Autodesk Inventor part; units mm, degrees
(part 3 of 6)
sketch "Sketch39" plane through (0, 0, 35) normal (0, 0, 1) x (1, 0, 0)
  line L0 (24.1, -52.4001) -> (24.1, -46.4001) projected
  line L1 (24.1, -90.2001) -> (30.1, -90.2001) projected
  line L2 (30.1, -46.4001) -> (30.1, -52.4001) projected
  line L3 (30.1, -96.2001) -> (24.1, -96.2001) projected
  line L4 (-30.1, -46.4001) -> (-24.1, -46.4001) projected
  line L5 (-24.1, -46.4001) -> (-24.1, -52.4001) projected
  line L6 (-24.1, -52.4001) -> (-30.1, -52.4001) projected
  line L7 (-30.1, -52.4001) -> (-30.1, -46.4001) projected
  line L8 (-30.1, -90.2001) -> (-24.1, -90.2001) projected
  line L9 (-24.1, -96.2001) -> (-30.1, -96.2001) projected
  line L10 (24.1, -46.4001) -> (30.1, -46.4001) projected
  line L11 (30.1, -52.4001) -> (24.1, -52.4001) projected
  line L12 (-44.1, -54.2001) -> (44.1, -54.2001) projected
  arc A0 (44.1, -64.2001) -> (44.1, -54.2001) centre (44.1, -59.2001) ccw projected
  line L13 (44.1, -64.2001) -> (44.1, -78.4001) projected
  arc A1 (44.1, -88.4001) -> (44.1, -78.4001) centre (44.1, -83.4001) ccw projected
  line L14 (44.1, -88.4001) -> (-44.1, -88.4001) projected
  line L15 (-44.1, -88.4001) -> (-44.1, -54.2001) projected
  line L16 (-103.1549, -6.3815) -> (-96.791, -0.0176) projected
  line L17 (-96.791, -0.0176) -> (-95.5889, 1.1845) projected
  line L18 (-95.5889, 1.1845) -> (-91.3463, -3.0581) projected
  line L19 (-91.3463, -3.0581) -> (-75.0828, -19.3216) projected
  line L20 (-75.0828, -19.3216) -> (-71.5473, -22.8571) projected
  line L21 (-71.5473, -22.8571) -> (-80.3154, -31.6252) projected
  line L22 (-80.3154, -31.6252) -> (-83.8509, -28.0897) projected
  line L23 (-83.8509, -28.0897) -> (-100.1144, -11.8263) projected
  line L24 (-100.1144, -11.8263) -> (-104.357, -7.5836) projected
  line L25 (-104.357, -7.5836) -> (-103.1549, -6.3815) projected
  line L26 (4.5, -160.1002) -> (-4.5, -160.1002) projected
  line L27 (-4.5, -160.1002) -> (-6.2, -160.1002) projected
  line L28 (-6.2, -160.1002) -> (-6.2, -154.1002) projected
  line L29 (-6.2, -154.1002) -> (-6.2, -131.1002) projected
  line L30 (-6.2, -131.1002) -> (-6.2, -126.1002) projected
  line L31 (-6.2, -126.1002) -> (6.2, -126.1002) projected
  line L32 (6.2, -126.1002) -> (6.2, -131.1002) projected
  line L33 (6.2, -131.1002) -> (6.2, -154.1002) projected
  line L34 (6.2, -154.1002) -> (6.2, -160.1002) projected
  line L35 (6.2, -160.1002) -> (4.5, -160.1002) projected
  line L36 (96.791, -0.0176) -> (103.1549, -6.3815) projected
  line L37 (103.1549, -6.3815) -> (104.357, -7.5836) projected
  line L38 (104.357, -7.5836) -> (100.1144, -11.8263) projected
  line L39 (100.1144, -11.8263) -> (83.8509, -28.0897) projected
  line L40 (83.8509, -28.0897) -> (80.3154, -31.6252) projected
  line L41 (80.3154, -31.6252) -> (71.5473, -22.8571) projected
  line L42 (71.5473, -22.8571) -> (75.0828, -19.3216) projected
  line L43 (75.0828, -19.3216) -> (91.3463, -3.0581) projected
  line L44 (91.3463, -3.0581) -> (95.5889, 1.1845) projected
  line L45 (95.5889, 1.1845) -> (96.791, -0.0176) projected
  line L46 (76.8724, -48.8001) -> (88.2822, -48.8001) projected
  line L47 (88.2822, -48.8001) -> (94.3529, -27.4901) projected
  line L48 (94.3529, -27.4901) -> (106.8333, -15.0097) projected
  arc A2 (106.8333, -15.0097) -> (88.1629, 3.6608) centre (97.4981, -5.6744) ccw projected
  line L49 (88.1629, 3.6608) -> (75.6824, -8.8196) projected
  line L50 (75.6824, -8.8196) -> (57.202, -21.3001) projected
  line L51 (57.202, -21.3001) -> (38.202, -31.3001) projected
  line L52 (38.202, -31.3001) -> (19.202, -21.3001) projected
  line L53 (19.202, -21.3001) -> (13.202, -3.65) projected
  line L54 (13.202, -3.65) -> (13.202, 14) projected
  arc A3 (13.202, 14) -> (-13.202, 14) centre (0, 14) ccw projected
  line L55 (-13.202, 14) -> (-13.202, -3.65) projected
  line L56 (-13.202, -3.65) -> (-19.202, -21.3001) projected
  line L57 (-19.202, -21.3001) -> (-38.202, -31.3001) projected
  line L58 (-38.202, -31.3001) -> (-57.202, -21.3001) projected
  line L59 (-57.202, -21.3001) -> (-75.6824, -8.8196) projected
  line L60 (-75.6824, -8.8196) -> (-88.1629, 3.6608) projected
  arc A4 (-88.1629, 3.6608) -> (-106.8333, -15.0097) centre (-97.4981, -5.6744) ccw projected
  line L61 (-106.8333, -15.0097) -> (-94.3529, -27.4901) projected
  line L62 (-94.3529, -27.4901) -> (-76.3482, -71.3001) projected
  line L63 (-76.3482, -71.3001) -> (-94.3529, -115.1101) projected
  line L64 (-94.3529, -115.1101) -> (-106.8333, -127.5905) projected
  arc A5 (-106.8333, -127.5905) -> (-88.1629, -146.2609) centre (-97.4981, -136.9257) ccw projected
  line L65 (-88.1629, -146.2609) -> (-75.6824, -133.7805) projected
  line L66 (-75.6824, -133.7805) -> (-57.202, -121.3001) projected
  line L67 (-57.202, -121.3001) -> (-38.202, -111.3001) projected
  line L68 (-38.202, -111.3001) -> (-19.202, -121.3001) projected
  line L69 (-19.202, -121.3001) -> (-13.202, -138.9501) projected
  line L70 (-13.202, -138.9501) -> (-13.202, -156.6002) projected
  arc A6 (-13.202, -156.6002) -> (13.202, -156.6002) centre (0, -156.6002) ccw projected
  line L71 (13.202, -156.6002) -> (13.202, -138.9501) projected
  line L72 (13.202, -138.9501) -> (19.202, -121.3001) projected
  line L73 (19.202, -121.3001) -> (38.202, -111.3001) projected
  line L74 (38.202, -111.3001) -> (57.202, -121.3001) projected
  line L75 (57.202, -121.3001) -> (75.6824, -133.7805) projected
  line L76 (75.6824, -133.7805) -> (88.1629, -146.2609) projected
  arc A7 (88.1629, -146.2609) -> (106.8333, -127.5905) centre (97.4981, -136.9257) ccw projected
  line L77 (106.8333, -127.5905) -> (94.3529, -115.1101) projected
  line L78 (94.3529, -115.1101) -> (88.2822, -93.8001) projected
  line L79 (88.2822, -93.8001) -> (76.8724, -93.8001) projected
  line L80 (76.8724, -93.8001) -> (76.8724, -48.8001) projected
  line L81 (-96.791, -142.5826) -> (-103.1549, -136.2186) projected
  line L82 (-103.1549, -136.2186) -> (-104.357, -135.0165) projected
  line L83 (-104.357, -135.0165) -> (-100.1144, -130.7739) projected
  line L84 (-100.1144, -130.7739) -> (-83.8509, -114.5104) projected
  line L85 (-83.8509, -114.5104) -> (-80.3154, -110.9749) projected
  line L86 (-80.3154, -110.9749) -> (-71.5473, -119.743) projected
  line L87 (-71.5473, -119.743) -> (-75.0828, -123.2786) projected
  line L88 (-75.0828, -123.2786) -> (-91.3463, -139.542) projected
  line L89 (-91.3463, -139.542) -> (-95.5889, -143.7847) projected
  line L90 (-95.5889, -143.7847) -> (-96.791, -142.5826) projected
  line L91 (103.1549, -136.2186) -> (96.791, -142.5826) projected
  line L92 (96.791, -142.5826) -> (95.5889, -143.7847) projected
  line L93 (95.5889, -143.7847) -> (91.3463, -139.542) projected
  line L94 (91.3463, -139.542) -> (75.0828, -123.2786) projected
  line L95 (75.0828, -123.2786) -> (71.5473, -119.743) projected
  line L96 (71.5473, -119.743) -> (80.3154, -110.9749) projected
  line L97 (80.3154, -110.9749) -> (83.8509, -114.5104) projected
  line L98 (83.8509, -114.5104) -> (100.1144, -130.7739) projected
  line L99 (100.1144, -130.7739) -> (104.357, -135.0165) projected
  line L100 (104.357, -135.0165) -> (103.1549, -136.2186) projected
  line L101 (-4.5, 17.5) -> (4.5, 17.5) projected
  line L102 (4.5, 17.5) -> (6.2, 17.5) projected
  line L103 (6.2, 17.5) -> (6.2, 11.5) projected
  line L104 (6.2, 11.5) -> (6.2, -11.5) projected
  line L105 (6.2, -11.5) -> (6.2, -16.5) projected
  line L106 (6.2, -16.5) -> (-6.2, -16.5) projected
  line L107 (-6.2, -16.5) -> (-6.2, -11.5) projected
  line L108 (-6.2, -11.5) -> (-6.2, 11.5) projected
  line L109 (-6.2, 11.5) -> (-6.2, 17.5) projected
  line L110 (-6.2, 17.5) -> (-4.5, 17.5) projected
  circle A8 centre (-27.1, -93.2001) radius 1.5
  circle A9 centre (-27.1, -49.4001) radius 1.5
  circle A10 centre (27.1, -93.2001) radius 1.5
  circle A11 centre (27.1, -49.4001) radius 1.5
  line L111 (30.1, -90.2001) -> (30.1, -96.2001) projected
  line L112 (24.1, -96.2001) -> (24.1, -90.2001) projected
  line L113 (-30.1, -96.2001) -> (-30.1, -90.2001) projected
  line L114 (-24.1, -90.2001) -> (-24.1, -96.2001) projected
  point P0 (0, 0)
  dimension "d566" = 3
  dimension "d567" = 3
  dimension "d568" = 3
  dimension "d569" = 3
  dimension "d570" = 3
  dimension "d571" = 3
  dimension "d572" = 3
  dimension "d575" = 3
  dimension "d576" = 3
  dimension "d577" = 3
  constraints: 4 centre point
  measures "d566" diameter of A8
  measures "d567" diameter of A9
  measures "d568" diameter of A10
  measures "d569" diameter of A11
  measures "d570" distance from line of L1 A10.centre
  measures "d571" distance from line of L10 A11.centre
  measures "d572" distance from line of L2 A10.centre
  measures "d575" distance from line of L8 A8.centre
  measures "d576" distance from line of L5 A9.centre
  measures "d577" distance from line of L4 A9.centre
extrude "Extrusion39" cut sketch "Sketch39" against normal blind 100 contours A8 | A9 | A10 | A11
sketch "Sketch40" plane through (0, 0, -5) normal (0, 0, -1) x (-1, 0, 0)
  circle A0 centre (-27.1, -49.4001) radius 1.5 projected
  circle A1 centre (-27.1, -93.2001) radius 1.5 projected
  circle A2 centre (27.1, -49.4001) radius 1.5 projected
  circle A3 centre (27.1, -93.2001) radius 1.5 projected
  line L0 (-3.1216, -126.8818) -> (-0.0216, -125.092) projected
  line L1 (-0.0216, -125.092) -> (3.0784, -126.8818) projected
  line L2 (3.0784, -126.8818) -> (3.0784, -130.4614) projected
  line L3 (3.0784, -130.4614) -> (-0.0216, -132.2511) projected
  line L4 (-0.0216, -132.2511) -> (-3.1216, -130.4614) projected
  line L5 (-3.1216, -130.4614) -> (-3.1216, -126.8818) projected
  line L6 (-3.2524, -13.9963) -> (-1.6252, -11.1823) projected
  line L7 (-1.6252, -11.1823) -> (1.6252, -11.1846) projected
  line L8 (1.6252, -11.1846) -> (3.2486, -14.0007) projected
  line L9 (3.2486, -14.0007) -> (1.6214, -16.8146) projected
  line L10 (1.6214, -16.8146) -> (-1.6291, -16.8124) projected
  line L11 (-1.6291, -16.8124) -> (-3.2524, -13.9963) projected
  line L12 (-76.9445, -120.8328) -> (-80.5331, -119.7332) projected
  line L13 (-80.5331, -119.7332) -> (-81.3752, -116.0755) projected
  line L14 (-81.3752, -116.0755) -> (-78.6286, -113.5175) projected
  line L15 (-78.6286, -113.5175) -> (-75.0399, -114.6171) projected
  line L16 (-75.0399, -114.6171) -> (-74.1979, -118.2748) projected
  line L17 (-74.1979, -118.2748) -> (-76.9445, -120.8328) projected
  line L18 (74.0578, -118.2007) -> (74.9468, -114.5542) projected
  line L19 (74.9468, -114.5542) -> (78.5493, -113.5008) projected
  line L20 (78.5493, -113.5008) -> (81.2629, -116.094) projected
  line L21 (81.2629, -116.094) -> (80.3739, -119.7405) projected
  line L22 (80.3739, -119.7405) -> (76.7714, -120.7939) projected
  line L23 (76.7714, -120.7939) -> (74.0578, -118.2007) projected
  line L24 (81.3332, -26.5207) -> (78.6197, -29.1139) projected
  line L25 (78.6197, -29.1139) -> (75.0172, -28.0605) projected
  line L26 (75.0172, -28.0605) -> (74.1282, -24.4139) projected
  line L27 (74.1282, -24.4139) -> (76.8417, -21.8207) projected
  line L28 (76.8417, -21.8207) -> (80.4442, -22.8741) projected
  line L29 (80.4442, -22.8741) -> (81.3332, -26.5207) projected
  line L30 (-76.9117, -21.8446) -> (-74.165, -24.4027) projected
  line L31 (-74.165, -24.4027) -> (-75.0071, -28.0604) projected
  line L32 (-75.0071, -28.0604) -> (-78.5957, -29.16) projected
  line L33 (-78.5957, -29.16) -> (-81.3424, -26.6019) projected
  line L34 (-81.3424, -26.6019) -> (-80.5003, -22.9442) projected
  line L35 (-80.5003, -22.9442) -> (-76.9117, -21.8446) projected
  circle A4 centre (-91.4877, -11.6848) radius 5 projected
  circle A5 centre (0, -148.1002) radius 5 projected
  circle A6 centre (91.4877, -11.6848) radius 5 projected
  circle A7 centre (91.4877, -130.9153) radius 5 projected
  circle A8 centre (-91.4877, -130.9153) radius 5 projected
  circle A9 centre (0, 5.5) radius 5 projected
  line L36 (-13.202, -3.65) -> (-19.202, -21.3001) projected
  line L37 (-19.202, -21.3001) -> (-38.202, -31.3001) projected
  line L38 (-38.202, -31.3001) -> (-57.202, -21.3001) projected
  line L39 (-57.202, -21.3001) -> (-75.6824, -8.8196) projected
  line L40 (-75.6824, -8.8196) -> (-88.1629, 3.6608) projected
  arc A10 (-88.1629, 3.6608) -> (-106.8333, -15.0097) centre (-97.4981, -5.6744) ccw projected
  line L41 (-106.8333, -15.0097) -> (-94.3529, -27.4901) projected
  line L42 (-94.3529, -27.4901) -> (-81.8724, -71.3001) projected
  line L43 (-81.8724, -71.3001) -> (-94.3529, -115.1101) projected
  line L44 (-94.3529, -115.1101) -> (-106.8333, -127.5905) projected
  arc A11 (-106.8333, -127.5905) -> (-88.1629, -146.2609) centre (-97.4981, -136.9257) ccw projected
  line L45 (-88.1629, -146.2609) -> (-75.6824, -133.7805) projected
  line L46 (-75.6824, -133.7805) -> (-57.202, -121.3001) projected
  line L47 (-57.202, -121.3001) -> (-38.202, -111.3001) projected
  line L48 (-38.202, -111.3001) -> (-19.202, -121.3001) projected
  line L49 (-19.202, -121.3001) -> (-13.202, -138.9501) projected
  line L50 (-13.202, -138.9501) -> (-13.202, -156.6002) projected
  arc A12 (-13.202, -156.6002) -> (13.202, -156.6002) centre (0, -156.6002) ccw projected
  line L51 (13.202, -156.6002) -> (13.202, -138.9501) projected
  line L52 (13.202, -138.9501) -> (19.202, -121.3001) projected
  line L53 (19.202, -121.3001) -> (38.202, -111.3001) projected
  line L54 (38.202, -111.3001) -> (57.202, -121.3001) projected
  line L55 (57.202, -121.3001) -> (75.6824, -133.7805) projected
  line L56 (75.6824, -133.7805) -> (88.1629, -146.2609) projected
  arc A13 (88.1629, -146.2609) -> (106.8333, -127.5905) centre (97.4981, -136.9257) ccw projected
  line L57 (106.8333, -127.5905) -> (94.3529, -115.1101) projected
  line L58 (94.3529, -115.1101) -> (76.3482, -71.3001) projected
  line L59 (76.3482, -71.3001) -> (94.3529, -27.4901) projected
  line L60 (94.3529, -27.4901) -> (106.8333, -15.0097) projected
  arc A14 (106.8333, -15.0097) -> (88.1629, 3.6608) centre (97.4981, -5.6744) ccw projected
  line L61 (88.1629, 3.6608) -> (75.6824, -8.8196) projected
  line L62 (75.6824, -8.8196) -> (57.202, -21.3001) projected
  line L63 (57.202, -21.3001) -> (38.202, -31.3001) projected
  line L64 (38.202, -31.3001) -> (19.202, -21.3001) projected
  line L65 (19.202, -21.3001) -> (13.202, -3.65) projected
  line L66 (13.202, -3.65) -> (13.202, 14) projected
  arc A15 (13.202, 14) -> (-13.202, 14) centre (0, 14) ccw projected
  line L67 (-13.202, 14) -> (-13.202, -3.65) projected
  line L68 (25.3102, -96.3001) -> (23.5204, -93.2001)
  line L69 (23.5204, -93.2001) -> (25.3102, -90.1001)
  line L70 (25.3102, -90.1001) -> (28.8898, -90.1001)
  line L71 (28.8898, -90.1001) -> (30.6796, -93.2001)
  line L72 (30.6796, -93.2001) -> (28.8898, -96.3001)
  line L73 (28.8898, -96.3001) -> (25.3102, -96.3001)
  line L74 (-28.8898, -90.1001) -> (-25.3102, -90.1001)
  line L75 (-25.3102, -90.1001) -> (-23.5204, -93.2001)
  line L76 (-23.5204, -93.2001) -> (-25.3102, -96.3001)
  line L77 (-25.3102, -96.3001) -> (-28.8898, -96.3001)
  line L78 (-28.8898, -96.3001) -> (-30.6796, -93.2001)
  line L79 (-30.6796, -93.2001) -> (-28.8898, -90.1001)
  line L80 (-28.8898, -52.5001) -> (-30.6796, -49.4001)
  line L81 (-30.6796, -49.4001) -> (-28.8898, -46.3001)
  line L82 (-28.8898, -46.3001) -> (-25.3102, -46.3001)
  line L83 (-25.3102, -46.3001) -> (-23.5204, -49.4001)
  line L84 (-23.5204, -49.4001) -> (-25.3102, -52.5001)
  line L85 (-25.3102, -52.5001) -> (-28.8898, -52.5001)
  line L86 (25.3102, -52.5001) -> (23.5204, -49.4001)
  line L87 (23.5204, -49.4001) -> (25.3102, -46.3001)
  line L88 (25.3102, -46.3001) -> (28.8898, -46.3001)
  line L89 (28.8898, -46.3001) -> (30.6796, -49.4001)
  line L90 (30.6796, -49.4001) -> (28.8898, -52.5001)
  line L91 (28.8898, -52.5001) -> (25.3102, -52.5001)
  line L92 (-3.1216, -126.8818) -> (-0.0216, -125.092) projected
  line L93 (-0.0216, -125.092) -> (3.0784, -126.8818) projected
  point P0 (0, 0)
  dimension "d580" = 3.1
  dimension "d581" = 3.1
  dimension "d582" = 3.1
  dimension "d583" = 3.1
  constraints: 48 end point, 4 coincident, 4 perpendicular, 52 other
  measures "d580" distance from line of L76 A1.centre
  measures "d581" distance from line of L69 A3.centre
  measures "d582" distance from line of L91 A2.centre
  measures "d583" distance from line of L82 A0.centre
extrude "Extrusion40" cut sketch "Sketch40" against normal blind 2.4 contours A0 | A1 | A2 | A3 | L68 L69 L70 L71 L72 L73 | L74 L75 L76 L77 L78 L79 | L80 L81 L82 L83 L84 L85 | L86 L87 L88 L89 L90 L91
sketch "Sketch41" plane through (76.8724, -93.8001, 10) normal (-1, 0, 0) x (0, 0, 1)
  arc A0 (2.2, 18.95) -> (6.3, 18.95) centre (4.25, 18.95) ccw projected
  line L0 (2.2, 18.95) -> (2.2, 25.95) projected
  arc A1 (6.3, 25.95) -> (2.2, 25.95) centre (4.25, 25.95) ccw projected
  line L1 (6.3, 25.95) -> (6.3, 18.95) projected
  line L2 (0, 0) -> (0, 45) projected
  line L3 (0, 0) -> (25, 0) projected
  line L4 (25, 45) -> (25, 0) projected
  line L5 (0, 45) -> (25, 45) projected
  circle A2 centre (20.5, 43.45) radius 1
  circle A3 centre (20.5, 1.45) radius 1
  circle A4 centre (3.5, 1.45) radius 1
  circle A5 centre (3.5, 43.45) radius 1
  circle A6 centre (12, 35.95) radius 8
  circle A7 centre (12, 8.95) radius 8
  circle A8 centre (12, 35.95) radius 8.15
  circle A9 centre (12, 8.95) radius 8.15
  point P0 (-10, 93.8001)
  dimension "d586" = 0.15
  dimension "d587" = 0.15
  constraints: 8 centre point, 12 other
  measures "d586" radial gap between concentric circles of A8 A6
  measures "d587" radial gap between concentric circles of A9 A7
extrude "Extrusion41" cut sketch "Sketch41" against normal blind 20 contours A2 | A3 | A4 | A5 | A6 | A7 | A8 | A9
ref_plane "Work Plane1" through (88.2822, -48.8001, 10) normal (1, 0, 0) x (0, 0, 1)
sketch "Sketch42" plane through (88.2822, -48.8001, 10) normal (1, 0, 0) x (0, 0, 1)
  circle A0 centre (20.5, 43.55) radius 1 projected
  circle A1 centre (12, 36.05) radius 8.15 projected
  circle A2 centre (3.5, 43.55) radius 1 projected
  line L0 (25, 22.5) -> (-15, 22.5) projected
  line L1 (25, 45) -> (25, 22.5) projected
  line L2 (0, 45) -> (25, 45) projected
  line L3 (0, 66.31) -> (0, 45) projected
  line L4 (-15, 66.31) -> (0, 66.31) projected
  line L5 (-15, 22.5) -> (-15, 66.31) projected
  circle A3 centre (12, 9.05) radius 8.15 projected
  circle A4 centre (3.5, 1.55) radius 1 projected
  circle A5 centre (20.5, 1.55) radius 1 projected
  line L6 (-15, -21.31) -> (0, -21.31) projected
  line L7 (0, 0) -> (0, -21.31) projected
  line L8 (0, 0) -> (25, 0) projected
  line L9 (25, 22.5) -> (25, 0) projected
  line L10 (25, 22.5) -> (-15, 22.5) projected
  line L11 (-15, -21.31) -> (-15, 22.5) projected
  line L12 (0, 0) -> (0, -21.31) projected
  line L13 (0, 0) -> (-15, 0)
  line L14 (0, 66.31) -> (0, 45) projected
  line L15 (0, 45) -> (-15, 45)
  line L16 (-15, 0) -> (25, 0)
  line L17 (25, 0) -> (25, 45)
  line L18 (25, 45) -> (-15, 45)
  line L19 (-15, 45) -> (-15, 0)
  point P0 (-10, -48.8001)
  constraints: 12 end point, 3 parallel, 2 perpendicular, 2 point on line, 1 horizontal
extrude "Extrusion42" add sketch "Sketch42" against normal blind 8 contours L9 L8 L13 L11 L0 | L0 L5 L15 L2 L1
hole "Hole6" at (0.0216, -156.6716, 19) at (-97.4593, -136.9463, 19) at (-97.5297, -5.6683, 19) at (0.0019, 14.0015, 19) at (97.5527, -5.7033, 19) at (97.5855, -136.9741, 19) direction (0, 0, -1) diameter 3 depth 6.5
sketch "Sketch43" plane through (0, 0, 10) normal (0, 0, 1) x (1, 0, 0)
  line L0 (30.1, -90.2001) -> (30.1, -96.2001) projected
  line L1 (30.1, -96.2001) -> (24.1, -96.2001) projected
  line L2 (24.1, -96.2001) -> (24.1, -90.2001) projected
  line L3 (24.1, -90.2001) -> (30.1, -90.2001) projected
  line L4 (-24.1, -52.4001) -> (-30.1, -52.4001) projected
  line L5 (-30.1, -52.4001) -> (-30.1, -46.4001) projected
  line L6 (-30.1, -46.4001) -> (-24.1, -46.4001) projected
  line L7 (-24.1, -46.4001) -> (-24.1, -52.4001) projected
  line L8 (-24.1, -96.2001) -> (-30.1, -96.2001) projected
  line L9 (-30.1, -96.2001) -> (-30.1, -90.2001) projected
  line L10 (-30.1, -90.2001) -> (-24.1, -90.2001) projected
  line L11 (-24.1, -90.2001) -> (-24.1, -96.2001) projected
  line L12 (30.1, -52.4001) -> (24.1, -52.4001) projected
  line L13 (24.1, -52.4001) -> (24.1, -46.4001) projected
  line L14 (24.1, -46.4001) -> (30.1, -46.4001) projected
  line L15 (30.1, -46.4001) -> (30.1, -52.4001) projected
  line L16 (-44.1, -88.4001) -> (-44.1, -54.2001) projected
  line L17 (-44.1, -54.2001) -> (44.1, -54.2001) projected
  arc A0 (44.1, -64.2001) -> (44.1, -54.2001) centre (44.1, -59.2001) ccw projected
  line L18 (44.1, -64.2001) -> (44.1, -78.4001) projected
  arc A1 (44.1, -88.4001) -> (44.1, -78.4001) centre (44.1, -83.4001) ccw projected
  line L19 (44.1, -88.4001) -> (-44.1, -88.4001) projected
  line L20 (-4.5, 17.5) -> (4.5, 17.5) projected
  line L21 (4.5, 17.5) -> (6.2, 17.5) projected
  line L22 (6.2, 17.5) -> (6.2, 11.5) projected
  line L23 (6.2, 11.5) -> (6.2, -11.5) projected
  line L24 (6.2, -11.5) -> (6.2, -16.5) projected
  line L25 (6.2, -16.5) -> (-6.2, -16.5) projected
  line L26 (-6.2, -16.5) -> (-6.2, -11.5) projected
  line L27 (-6.2, -11.5) -> (-6.2, 11.5) projected
  line L28 (-6.2, 11.5) -> (-6.2, 17.5) projected
  line L29 (-6.2, 17.5) -> (-4.5, 17.5) projected
  line L30 (4.5, -160.1002) -> (-4.5, -160.1002) projected
  line L31 (-4.5, -160.1002) -> (-6.2, -160.1002) projected
  line L32 (-6.2, -160.1002) -> (-6.2, -154.1002) projected
  line L33 (-6.2, -154.1002) -> (-6.2, -131.1002) projected
  line L34 (-6.2, -131.1002) -> (-6.2, -126.1002) projected
  line L35 (-6.2, -126.1002) -> (6.2, -126.1002) projected
  line L36 (6.2, -126.1002) -> (6.2, -131.1002) projected
  line L37 (6.2, -131.1002) -> (6.2, -154.1002) projected
  line L38 (6.2, -154.1002) -> (6.2, -160.1002) projected
  line L39 (6.2, -160.1002) -> (4.5, -160.1002) projected
  line L40 (-103.1549, -6.3815) -> (-96.791, -0.0176) projected
  line L41 (-96.791, -0.0176) -> (-95.5889, 1.1845) projected
  line L42 (-95.5889, 1.1845) -> (-91.3463, -3.0581) projected
  line L43 (-91.3463, -3.0581) -> (-75.0828, -19.3216) projected
  line L44 (-75.0828, -19.3216) -> (-71.5473, -22.8571) projected
  line L45 (-71.5473, -22.8571) -> (-80.3154, -31.6252) projected
  line L46 (-80.3154, -31.6252) -> (-83.8509, -28.0897) projected
  line L47 (-83.8509, -28.0897) -> (-100.1144, -11.8263) projected
  line L48 (-100.1144, -11.8263) -> (-104.357, -7.5836) projected
  line L49 (-104.357, -7.5836) -> (-103.1549, -6.3815) projected
  line L50 (96.791, -0.0176) -> (103.1549, -6.3815) projected
  line L51 (103.1549, -6.3815) -> (104.357, -7.5836) projected
  line L52 (104.357, -7.5836) -> (100.1144, -11.8263) projected
  line L53 (100.1144, -11.8263) -> (83.8509, -28.0897) projected
  line L54 (83.8509, -28.0897) -> (80.3154, -31.6252) projected
  line L55 (80.3154, -31.6252) -> (71.5473, -22.8571) projected
  line L56 (71.5473, -22.8571) -> (75.0828, -19.3216) projected
  line L57 (75.0828, -19.3216) -> (91.3463, -3.0581) projected
  line L58 (91.3463, -3.0581) -> (95.5889, 1.1845) projected
  line L59 (95.5889, 1.1845) -> (96.791, -0.0176) projected
  line L60 (103.1549, -136.2186) -> (96.791, -142.5826) projected
  line L61 (96.791, -142.5826) -> (95.5889, -143.7847) projected
  line L62 (95.5889, -143.7847) -> (91.3463, -139.542) projected
  line L63 (91.3463, -139.542) -> (75.0828, -123.2786) projected
  line L64 (75.0828, -123.2786) -> (71.5473, -119.743) projected
  line L65 (71.5473, -119.743) -> (80.3154, -110.9749) projected
  line L66 (80.3154, -110.9749) -> (83.8509, -114.5104) projected
  line L67 (83.8509, -114.5104) -> (100.1144, -130.7739) projected
  line L68 (100.1144, -130.7739) -> (104.357, -135.0165) projected
  line L69 (104.357, -135.0165) -> (103.1549, -136.2186) projected
  line L70 (-96.791, -142.5826) -> (-103.1549, -136.2186) projected
  line L71 (-103.1549, -136.2186) -> (-104.357, -135.0165) projected
  line L72 (-104.357, -135.0165) -> (-100.1144, -130.7739) projected
  line L73 (-100.1144, -130.7739) -> (-83.8509, -114.5104) projected
  line L74 (-83.8509, -114.5104) -> (-80.3154, -110.9749) projected
  line L75 (-80.3154, -110.9749) -> (-71.5473, -119.743) projected
  line L76 (-71.5473, -119.743) -> (-75.0828, -123.2786) projected
  line L77 (-75.0828, -123.2786) -> (-91.3463, -139.542) projected
  line L78 (-91.3463, -139.542) -> (-95.5889, -143.7847) projected
  line L79 (-95.5889, -143.7847) -> (-96.791, -142.5826) projected
  line L80 (76.8724, -48.8001) -> (88.2822, -48.8001) projected
  line L81 (88.2822, -48.8001) -> (94.3529, -27.4901) projected
  line L82 (94.3529, -27.4901) -> (106.8333, -15.0097) projected
  arc A2 (106.8333, -15.0097) -> (88.1629, 3.6608) centre (97.4981, -5.6744) ccw projected
  line L83 (88.1629, 3.6608) -> (75.6824, -8.8196) projected
  line L84 (75.6824, -8.8196) -> (57.202, -21.3001) projected
  line L85 (57.202, -21.3001) -> (38.202, -31.3001) projected
  line L86 (38.202, -31.3001) -> (19.202, -21.3001) projected
  line L87 (19.202, -21.3001) -> (13.202, -3.65) projected
  line L88 (13.202, -3.65) -> (13.202, 14) projected
  arc A3 (13.202, 14) -> (-13.202, 14) centre (0, 14) ccw projected
  line L89 (-13.202, 14) -> (-13.202, -3.65) projected
  line L90 (-13.202, -3.65) -> (-19.202, -21.3001) projected
  line L91 (-19.202, -21.3001) -> (-38.202, -31.3001) projected
  line L92 (-38.202, -31.3001) -> (-57.202, -21.3001) projected
  line L93 (-57.202, -21.3001) -> (-75.6824, -8.8196) projected
  line L94 (-75.6824, -8.8196) -> (-88.1629, 3.6608) projected
  arc A4 (-88.1629, 3.6608) -> (-106.8333, -15.0097) centre (-97.4981, -5.6744) ccw projected
  line L95 (-106.8333, -15.0097) -> (-94.3529, -27.4901) projected
  line L96 (-94.3529, -27.4901) -> (-76.3482, -71.3001) projected
  line L97 (-76.3482, -71.3001) -> (-94.3529, -115.1101) projected
  line L98 (-94.3529, -115.1101) -> (-106.8333, -127.5905) projected
  arc A5 (-106.8333, -127.5905) -> (-88.1629, -146.2609) centre (-97.4981, -136.9257) ccw projected
  line L99 (-88.1629, -146.2609) -> (-75.6824, -133.7805) projected
  line L100 (-75.6824, -133.7805) -> (-57.202, -121.3001) projected
  line L101 (-57.202, -121.3001) -> (-38.202, -111.3001) projected
  line L102 (-38.202, -111.3001) -> (-19.202, -121.3001) projected
  line L103 (-19.202, -121.3001) -> (-13.202, -138.9501) projected
  line L104 (-13.202, -138.9501) -> (-13.202, -156.6002) projected
  arc A6 (-13.202, -156.6002) -> (13.202, -156.6002) centre (0, -156.6002) ccw projected
  line L105 (13.202, -156.6002) -> (13.202, -138.9501) projected
  line L106 (13.202, -138.9501) -> (19.202, -121.3001) projected
  line L107 (19.202, -121.3001) -> (38.202, -111.3001) projected
  line L108 (38.202, -111.3001) -> (57.202, -121.3001) projected
  line L109 (57.202, -121.3001) -> (75.6824, -133.7805) projected
  line L110 (75.6824, -133.7805) -> (88.1629, -146.2609) projected
  arc A7 (88.1629, -146.2609) -> (106.8333, -127.5905) centre (97.4981, -136.9257) ccw projected
  line L111 (106.8333, -127.5905) -> (94.3529, -115.1101) projected
  line L112 (94.3529, -115.1101) -> (88.2822, -93.8001) projected
  line L113 (88.2822, -93.8001) -> (76.8724, -93.8001) projected
  line L114 (76.8724, -93.8001) -> (76.8724, -48.8001) projected
  line L115 (0, -16.5) -> (0, -31.5)
  line L116 (-75.9313, -27.2412) -> (-65.3247, -37.8478)
  line L117 (-75.9313, -115.359) -> (-65.3247, -104.7524)
  line L118 (0, -126.1002) -> (0, -111.1002)
  line L119 (75.9313, -27.2412) -> (65.3247, -37.8478)
  line L120 (75.9313, -115.359) -> (65.3247, -104.7524)
  line L121 (65.3247, -37.8478) -> (69.974, -42.497)
  line L122 (65.3247, -37.8478) -> (60.6755, -33.1986)
  line L123 (69.974, -42.497) -> (60.6755, -33.1986)
  line L124 (60.6755, -33.1986) -> (56.0263, -37.8478)
  line L125 (56.0263, -37.8478) -> (65.3247, -47.1462)
  line L126 (65.3247, -47.1462) -> (69.974, -42.497)
  line L127 (0, -31.5) -> (6.575, -31.5)
  line L128 (0, -31.5) -> (-6.575, -31.5)
  line L129 (-65.3247, -37.8478) -> (-60.6755, -33.1986)
  line L130 (-60.6755, -33.1986) -> (-65.3247, -37.8478)
  line L131 (-69.974, -42.497) -> (-65.3247, -37.8478)
  line L132 (-65.3247, -104.7524) -> (-60.6755, -109.4016)
  line L133 (-65.3247, -104.7524) -> (-69.974, -100.1031)
  line L134 (0, -111.1002) -> (6.575, -111.1002)
  line L135 (0, -111.1002) -> (-6.575, -111.1002)
  line L136 (65.3247, -104.7524) -> (60.6755, -109.4016)
  line L137 (65.3247, -104.7524) -> (69.974, -100.1031)
  line L138 (60.6755, -109.4016) -> (69.974, -100.1031)
  line L139 (69.974, -100.1031) -> (65.3247, -95.4539)
  line L140 (65.3247, -95.4539) -> (56.0263, -104.7524)
  line L141 (56.0263, -104.7524) -> (60.6755, -109.4016)
  line L142 (-6.575, -111.1002) -> (6.575, -111.1002)
  line L143 (6.575, -111.1002) -> (6.575, -104.5252)
  line L144 (6.575, -104.5252) -> (-6.575, -104.5252)
  line L145 (-6.575, -104.5252) -> (-6.575, -111.1002)
  line L146 (-69.974, -100.1031) -> (-60.6755, -109.4016)
  line L147 (-60.6755, -109.4016) -> (-56.0263, -104.7524)
  line L148 (-56.0263, -104.7524) -> (-65.3247, -95.4539)
  line L149 (-65.3247, -95.4539) -> (-69.974, -100.1031)
  line L150 (-69.974, -42.497) -> (-60.6755, -33.1986)
  line L151 (-60.6755, -33.1986) -> (-56.0263, -37.8478)
  line L152 (-56.0263, -37.8478) -> (-65.3247, -47.1462)
  line L153 (-65.3247, -47.1462) -> (-69.974, -42.497)
  line L154 (6.575, -31.5) -> (-6.575, -31.5)
  line L155 (-6.575, -31.5) -> (-6.575, -38.075)
  line L156 (-6.575, -38.075) -> (6.575, -38.075)
  line L157 (6.575, -38.075) -> (6.575, -31.5)
  point P0 (0, 0)
  dimension "d599" = 15
  dimension "d600" = 15
  dimension "d602" = 15
  dimension "d603" = 15
  dimension "d605" = 15
  dimension "d606" = 90
  dimension "d607" = 90
  dimension "d608" = 90
  dimension "d609" = 90
  dimension "d611" = 15
  dimension "d612" = 6.575
  dimension "d616" = 6.575
  dimension "d618" = 90
  dimension "d619" = 90
  dimension "d620" = 6.575
  dimension "d621" = 6.575
  dimension "d622" = 6.575
  dimension "d625" = 6.575
  dimension "d626" = 6.575
  dimension "d627" = 90
  dimension "d628" = 6.575
  dimension "d629" = 6.575
  dimension "d630" = 6.575
  dimension "d631" = 6.575
  dimension "d632" = 90
  dimension "d633" = 90
  dimension "d638" = 90
  dimension "d639" = 90
  dimension "d640" = 6.575
  dimension "d641" = 6.575
  dimension "d644" = 6.575
  dimension "d647" = 6.575
  dimension "d648" = 6.575
  dimension "d683" = 6.575
  dimension "d684" = 6.575
  dimension "d685" = 19.777
  constraints: 86 end point, 13 parallel, 6 horizontal, 6 midpoint, 6 perpendicular, 3 collinear, 2 point on line, 2 vertical
  measures "d599" distance of L115.start L115.end
  measures "d600" distance of L116.start L116.end
  measures "d602" distance of L117.start L117.end
  measures "d603" distance of L118.start L118.end
  measures "d605" distance of L119.start L119.end
  measures "d606" angle of L119 L55
  measures "d607" angle of L45 L116
  measures "d608" angle of L117 L75
  measures "d609" angle of L65 L120
  measures "d611" distance of L120.start L120.end
  measures "d612" distance of L119.end L121.end
  measures "d616" distance of L119.end L122.end
  measures "d618" angle of L119 L121
  measures "d619" angle of L119 L122
  measures "d620" distance of L124.end L122.end
  measures "d621" distance of L115.end L127.end
  measures "d622" distance of L115.end L128.end
  measures "d625" distance of L129.end L116.end
  measures "d626" distance of L131.start L116.end
  measures "d627" angle of L131 L116
  measures "d628" distance of L117.end L132.end
  measures "d629" distance of L117.end L133.end
  measures "d630" distance of L118.end L134.end
  measures "d631" distance of L118.end L135.end
  measures "d632" angle of L117 L133
  measures "d633" angle of L117 L132
  measures "d638" angle of L136 L120
  measures "d639" angle of L120 L137
  measures "d640" distance of L140.end L138.start
  measures "d641" distance of L134.end L143.end
  measures "d644" distance of L132.end L147.end
  measures "d647" distance of L129.end L151.end
  measures "d648" distance of L128.end L155.end
  measures "d683" distance from line of L141 L120.end
  measures "d684" distance from line of L139 L120.end
  measures "d685" distance from line of L136.end L111
extrude "Extrusion43" add sketch "Sketch43" along normal blind 6 contours L121 L126 L125 L124 L122 | L127 L157 L156 L155 L128 | L129 L151 L152 L153 L131 | L133 L149 L148 L147 L132 | L135 L145 L144 L143 L134 | L136 L141 L140 L139 L137
chamfer "Chamfer12" distance 10 angle 45 1 edges at (-44.1, -71.3001, 10)
sketch "Sketch46" plane through (0, 0, 14) normal (0, 0, -1) x (-1, 0, 0)
  circle A0 centre (-0.0019, 14.0015) radius 1.5 projected
  line L0 (3.0981, 15.7913) -> (3.0981, 12.2117)
  line L1 (3.0981, 12.2117) -> (-0.0019, 10.422)
  line L2 (-0.0019, 10.422) -> (-3.1019, 12.2117)
  line L3 (-3.1019, 12.2117) -> (-3.1019, 15.7913)
  line L4 (-3.1019, 15.7913) -> (-0.0019, 17.5811)
  line L5 (-0.0019, 17.5811) -> (3.0981, 15.7913)
  circle A1 centre (97.5297, -5.6683) radius 1.5 projected
  line L6 (100.0608, -3.1372) -> (100.9873, -6.5948)
  line L7 (100.9873, -6.5948) -> (98.4562, -9.1259)
  line L8 (98.4562, -9.1259) -> (94.9986, -8.1995)
  line L9 (94.9986, -8.1995) -> (94.0721, -4.7419)
  line L10 (94.0721, -4.7419) -> (96.6032, -2.2107)
  line L11 (96.6032, -2.2107) -> (100.0608, -3.1372)
  circle A2 centre (97.4593, -136.9463) radius 1.5 projected
  line L12 (99.9905, -139.4775) -> (96.5329, -140.4039)
  line L13 (96.5329, -140.4039) -> (94.0017, -137.8728)
  line L14 (94.0017, -137.8728) -> (94.9282, -134.4152)
  line L15 (94.9282, -134.4152) -> (98.3858, -133.4887)
  line L16 (98.3858, -133.4887) -> (100.9169, -136.0199)
  line L17 (100.9169, -136.0199) -> (99.9905, -139.4775)
  circle A3 centre (-0.0216, -156.6716) radius 1.5 projected
  line L18 (-0.0216, -160.2511) -> (-3.1216, -158.4614)
  line L19 (-3.1216, -158.4614) -> (-3.1216, -154.8818)
  line L20 (-3.1216, -154.8818) -> (-0.0216, -153.092)
  line L21 (-0.0216, -153.092) -> (3.0784, -154.8818)
  line L22 (3.0784, -154.8818) -> (3.0784, -158.4614)
  line L23 (3.0784, -158.4614) -> (-0.0216, -160.2511)
  circle A4 centre (-97.5855, -136.9741) radius 1.5 projected
  line L24 (-96.6591, -140.4317) -> (-100.1167, -139.5053)
  line L25 (-100.1167, -139.5053) -> (-101.0431, -136.0477)
  line L26 (-101.0431, -136.0477) -> (-98.512, -133.5165)
  line L27 (-98.512, -133.5165) -> (-95.0544, -134.443)
  line L28 (-95.0544, -134.443) -> (-94.1279, -137.9006)
  line L29 (-94.1279, -137.9006) -> (-96.6591, -140.4317)
  circle A5 centre (-97.5527, -5.7033) radius 1.5 projected
  line L30 (-94.0951, -4.7768) -> (-95.0215, -8.2344)
  line L31 (-95.0215, -8.2344) -> (-98.4792, -9.1609)
  line L32 (-98.4792, -9.1609) -> (-101.0103, -6.6298)
  line L33 (-101.0103, -6.6298) -> (-100.0838, -3.1722)
  line L34 (-100.0838, -3.1722) -> (-96.6262, -2.2457)
  line L35 (-96.6262, -2.2457) -> (-94.0951, -4.7768)
  line L36 (-6.2, -11.5) -> (6.2, -11.5) projected
  line L37 (75.0828, -19.3216) -> (83.8509, -28.0897) projected
  line L38 (83.8509, -114.5104) -> (75.0828, -123.2786) projected
  line L39 (6.2, -131.1002) -> (-6.2, -131.1002) projected
  line L40 (-75.0828, -123.2786) -> (-83.8509, -114.5104) projected
  line L41 (-83.8509, -28.0897) -> (-75.0828, -19.3216) projected
  point P0 (0, 0)
  dimension "d663" = 3.1
  dimension "d664" = 3.1
  dimension "d665" = 3.1
  dimension "d666" = 3.1
  dimension "d667" = 3.1
  dimension "d668" = 3.1
  constraints: 72 end point, 6 coincident, 6 perpendicular, 78 other
  measures "d663" distance from line of L1 point (-0.002, 14.002)
  measures "d664" distance from line of L30 point (-97.553, -5.703)
  measures "d665" distance from line of L28 point (-97.586, -136.974)
  measures "d666" distance from line of L21 A3.centre
  measures "d667" distance from line of L13 point (97.459, -136.946)
  measures "d668" distance from line of L7 point (97.53, -5.668)
extrude "Extrusion46" cut sketch "Sketch46" against normal blind 2.4 contours A0 | L0 L1 L2 L3 L4 L5 | A1 | L6 L7 L8 L9 L10 L11 | A2 | L12 L13 L14 L15 L16 L17 | A3 | L18 L19 L20 L21 L22 L23 | A4 | L24 L25 L26 L27 L28 L29 | A5 | L30 L31 L32 L33 L34 L35
sketch "Sketch47" plane through (-6.575, -111.1002, 10) normal (0, -1, 0) x (1, 0, 0)
  line L0 (0, 0) -> (13.15, 0) projected
  line L1 (0, 0) -> (0, 6) projected
  line L2 (13.15, 6) -> (0, 6) projected
  line L3 (13.15, 0) -> (13.15, 6) projected
  line L4 (2, 0) -> (11.15, 0)
  line L5 (11.15, 0) -> (11.15, 4)
  line L6 (11.15, 4) -> (2, 4)
  line L7 (2, 4) -> (2, 0)
  point P0 (6.575, -10)
  point P1 (6.575, 0)
  point P2 (6.575, 0)
  dimension "d671" = 9.15
  dimension "d672" = 4
  constraints: 8 end point, 2 coincident, 2 midpoint, 2 parallel, 1 horizontal, 1 perpendicular
  measures "d671" distance of L4.start L4.end
  measures "d672" distance of L6.end L4.start
extrude "Extrusion47" cut sketch "Sketch47" against normal up to surface (79.6002 mm away) contours L7 L6 L5 L0
sketch "Sketch48" plane through (60.6755, -33.1986, 10) normal (0.7071068, 0.7071068, 0) x (-0.7071068, 0.7071068, 0)
  line L0 (-2, 0) -> (-11.15, 0)
  line L1 (-11.15, 0) -> (-11.15, 4)
  line L2 (-11.15, 4) -> (-2, 4)
  line L3 (-2, 4) -> (-2, 0)
  line L4 (-13.15, 0) -> (0, 0) projected
  line L5 (-13.15, 0) -> (-13.15, 6) projected
  line L6 (0, 6) -> (-13.15, 6) projected
  line L7 (0, 0) -> (0, 6) projected
  point P0 (66.379, -10)
  point P1 (-6.575, 0)
  point P2 (-6.575, 0)
  dimension "d675" = 4
  dimension "d676" = 9.15
  constraints: 8 end point, 2 coincident, 2 midpoint, 2 parallel, 1 horizontal, 1 perpendicular
  measures "d675" distance of L2.end L0.start
  measures "d676" distance of L1.end L2.end
extrude "Extrusion48" cut sketch "Sketch48" against normal up to surface (6.575 mm away) contours L0 L1 L2 L3
sketch "Sketch49" plane through (69.974, -100.1031, 16) normal (0.7071068, -0.7071068, 0) x (-0.7071068, -0.7071068, 0)
  line L0 (13.15, 6) -> (0, 6) projected
  line L1 (13.15, 6) -> (13.15, 0) projected
  line L2 (0, 0) -> (13.15, 0) projected
  line L3 (0, 6) -> (0, 0) projected
  line L4 (11.15, 2) -> (2, 2)
  line L5 (2, 2) -> (2, 6)
  line L6 (2, 6) -> (11.15, 6)
  line L7 (11.15, 6) -> (11.15, 2)
  point P0 (-21.3045, 16)
  point P1 (6.575, 6)
  point P2 (6.575, 6)
  point P3 (11.15, 6)
  point P4 (2, 6)
  dimension "d679" = 4
  dimension "d680" = 9.15
  constraints: 8 end point, 2 coincident, 2 midpoint, 2 parallel, 1 horizontal, 1 perpendicular
  measures "d679" distance of L4.end L5.end
  measures "d680" distance of L4.start L4.end
extrude "Extrusion49" cut sketch "Sketch49" against normal up to surface (6.575 mm away) contours L7 L4 L5 L0
sketch "Sketch50" plane through (-60.6755, -109.4016, 16) normal (-0.7071068, -0.7071068, 0) x (-0.7071068, 0.7071068, 0)
  line L0 (13.15, 6) -> (0, 6) projected
  line L1 (13.15, 6) -> (13.15, 0) projected
  line L2 (0, 0) -> (13.15, 0) projected
  line L3 (0, 6) -> (0, 0) projected
  line L4 (11.15, 6) -> (2, 6)
  line L5 (2, 6) -> (2, 2)
  line L6 (2, 2) -> (11.15, 2)
  line L7 (11.15, 2) -> (11.15, 6)
  point P0 (34.4545, 16)
  point P1 (6.575, 6)
  point P2 (6.575, 6)
  point P3 (11.15, 6)
  point P4 (2, 6)
  dimension "d686" = 4
  dimension "d687" = 9.15
  constraints: 8 end point, 2 coincident, 2 midpoint, 2 parallel, 1 horizontal, 1 perpendicular
  measures "d686" distance of L4.end L5.end
  measures "d687" distance of L5.end L6.end
extrude "Extrusion50" cut sketch "Sketch50" against normal up to surface (6.575 mm away) contours L7 L6 L5 L0
sketch "Sketch51" plane through (-69.974, -42.497, 10) normal (-0.7071068, 0.7071068, 0) x (-0.7071068, -0.7071068, 0)
  line L0 (-2, 4) -> (-11.15, 4)
  line L1 (-11.15, 4) -> (-11.15, 0)
  line L2 (-11.15, 0) -> (-2, 0)
  line L3 (-2, 0) -> (-2, 4)
  line L4 (-13.15, 0) -> (0, 0) projected
  line L5 (-13.15, 0) -> (-13.15, 6) projected
  line L6 (0, 6) -> (-13.15, 6) projected
  line L7 (0, 0) -> (0, 6) projected
  point P0 (-79.529, -10)
  point P1 (-6.575, 0)
  point P2 (-6.575, 0)
  dimension "d690" = 4
  dimension "d691" = 9.15
  constraints: 8 end point, 2 coincident, 2 midpoint, 2 parallel, 1 horizontal, 1 perpendicular
  measures "d690" distance of L0.end L1.end
  measures "d691" distance of L0.start L0.end
extrude "Extrusion51" cut sketch "Sketch51" against normal up to surface (6.575 mm away) contours L3 L2 L1 L0
sketch "Sketch52" plane through (-30.1, -96.2001, 10) normal (-1, 0, 0) x (0, 0, 1)
  line L0 (0, 0) -> (0, 6) projected
  line L1 (0, 0) -> (25, 0) projected
  line L2 (25, 49.8) -> (25, 0) projected
  line L3 (0, 49.8) -> (25, 49.8) projected
  line L4 (0, 43.8) -> (0, 49.8) projected
  line L5 (0, 43.8) -> (15, 43.8) projected
  line L6 (15, 6) -> (15, 43.8) projected
  line L7 (0, 6) -> (15, 6) projected
  point P0 (-10, 96.2001)
extrude "Extrusion52" cut sketch "Sketch52" against normal up to surface (60.2 mm away)
chamfer "Chamfer13" distance 4.75 distance2 10 1 edges at (99.973, -139.4006, 10) measured on face at (67.5067, -74.7424, 10)
chamfer "Chamfer14" distance 4.75 distance2 10 1 edges at (0, -160.1002, 10) measured on face at (67.5067, -74.7424, 10)
chamfer "Chamfer15" distance 4.75 distance2 10 1 edges at (-99.973, -3.1996, 10) measured on face at (67.5067, -74.7424, 10)
chamfer "Chamfer16" distance 4.75 distance2 10 1 edges at (-99.973, -139.4006, 10) measured on face at (67.5067, -74.7424, 10)
chamfer "Chamfer17" distance 4.75 distance2 10 1 edges at (0, 17.5, 10) measured on face at (67.5067, -74.7424, 10)
chamfer "Chamfer18" distance 4.75 distance2 10 1 edges at (99.973, -3.1996, 10) measured on face at (67.5067, -74.7424, 10)
sketch "Sketch53" plane through (0, 0, 35) normal (0, 0, 1) x (1, 0, 0)
  line L0 (88.2822, -48.8001) -> (76.8724, -48.8001) projected
  line L1 (76.8724, -48.8001) -> (76.8724, -93.8001) projected
  line L2 (76.8724, -93.8001) -> (88.2822, -93.8001) projected
  line L3 (88.2822, -48.8001) -> (88.2822, -93.8001) projected
  line L4 (88.2822, -93.8001) -> (94.3529, -115.1101) projected
  line L5 (88.2822, -93.8001) -> (84.2822, -93.8001)
  line L6 (84.2822, -93.8001) -> (84.2822, -48.8001)
  line L7 (84.2822, -48.8001) -> (88.2822, -48.8001)
  line L8 (88.2822, -48.8001) -> (88.2822, -93.8001)
  point P0 (0, 0)
  dimension "d714" = 4
  constraints: 8 end point, 2 parallel, 1 horizontal, 1 perpendicular, 1 point on line
  measures "d714" distance of L5.end L2.end
extrude "Extrusion53" cut sketch "Sketch53" against normal up to surface (25 mm away) contours L6 L2 L1 L0
sketch "Sketch54" plane through (88.2822, -48.8001, 10) normal (1, 0, 0) x (0, 0, -1)
  line L0 (-6, -19.05) -> (-6, -26.05)
  arc A0 (-2.5, -19.05) -> (-6, -19.05) centre (-4.25, -19.05) ccw
  line L1 (-2.5, -26.05) -> (-2.5, -19.05)
  arc A1 (-6, -26.05) -> (-2.5, -26.05) centre (-4.25, -26.05) ccw
  line L2 (-6.15, -26.05) -> (-6.15, -19.05)
  arc A2 (-2.35, -19.05) -> (-6.15, -19.05) centre (-4.25, -19.05) ccw
  line L3 (-2.35, -19.05) -> (-2.35, -26.05)
  arc A3 (-6.15, -26.05) -> (-2.35, -26.05) centre (-4.25, -26.05) ccw
  point P0 (10, 48.8001)
  dimension "d717" = 0.15
  constraints: 8 end point, 8 point on circle, 4 centre point, 2 vertical, 11 other
  measures "d717" distance between parallel lines of L2 L0
extrude "Extrusion54" cut sketch "Sketch54" against normal blind 10.25 contours A0 L1 A1 L0 | L2 A2 L3 A3